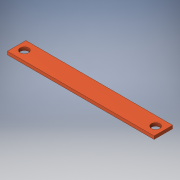
# Autodesk Inventor part: CU4
Saved by Autodesk Inventor 2016 (Build 200138000, 138)
## iProperties
Created: 2018-04-30
Part Number: CU4
Material: Copper
Document SubType Name: Modeling
Designer: Phil Erle
Density: 8.94 g/cm^3
Appearance: Copper - Satin
Author: Phil Erle
Autodesk Inventor part; units mm, degrees
ref_plane "YZ Plane" through (0, 0, 0) normal (1, 0, 0) x (0, 1, 0)
ref_plane "XZ Plane" through (0, 0, 0) normal (0, 1, 0) x (-1, 0, 0)
ref_plane "XY Plane" through (0, 0, 0) normal (0, 0, 1) x (1, 0, 0)
sketch "Sketch1" plane through (0, 0, 0) normal (0, 0, 1) x (1, 0, 0)
  line L0 (-47.5, -6) -> (47.5, -6)
  line L1 (47.5, -6) -> (47.5, 6)
  line L2 (47.5, 6) -> (-47.5, 6)
  line L3 (-47.5, 6) -> (-47.5, -6)
  line L4 (-47.5, -6) -> (47.5, 6) construction
  line L5 (47.5, -6) -> (-47.5, 6) construction
  point P0 (0, 0)
  dimension "d0" = 95
  dimension "d1" = 12
  constraints: 12 end point, 2 midpoint, 2 parallel, 1 horizontal, 1 perpendicular
  measures "d0" distance of L2.end L1.end
  measures "d1" distance of L1.end L0.end
extrude "Extrusion1" add sketch "Sketch1" along normal blind 2
sketch "Sketch2" plane through (0, 0, 2) normal (0, 0, 1) x (1, 0, 0)
  line L0 (-42.5, 0) -> (42.5, 0) construction
  point P0 (0, 0)
  point P1 (0, 0)
  dimension "d4" = 85
  constraints: 3 coincident, 2 end point, 1 horizontal, 1 horizontal alignment, 1 midpoint
  measures "d4" distance of L0.start L0.end
hole "Hole1" at (-42.5, 0, 2) at (42.5, 0, 2) direction (0, 0, -1) diameter 5.5 depth 8 tip angle 118 clearance for "Countersunk Flat Head Screw DIN EN ISO 2009" size "M5" standard "DIN"
body "Solid1"
